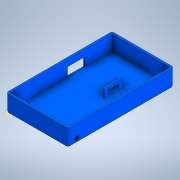
# Autodesk Inventor part: OuterCase
Saved by Autodesk Inventor 2021 (Build 250183000, 183)
## iProperties
Created: 2021-01-18
Part Number: OuterCase
Material: Generic
Document SubType Name: Modeling
Designer: Jayan
Density: 1 g/cm^3
Appearance: Default
Author: Jayan
Autodesk Inventor part; units mm, degrees
ref_plane "YZ Plane" through (0, 0, 0) normal (1, 0, 0) x (0, 1, 0)
ref_plane "XZ Plane" through (0, 0, 0) normal (0, 1, 0) x (-1, 0, 0)
ref_plane "XY Plane" through (0, 0, 0) normal (0, 0, 1) x (1, 0, 0)
sketch "Sketch1" plane through (0, 0, 0) normal (0, 1, 0) x (-1, 0, 0)
  line L0 (0, 0) -> (88.9, 0)
  line L1 (88.9, 0) -> (88.9, -152.4)
  line L2 (88.9, -152.4) -> (0, -152.4)
  line L3 (0, -152.4) -> (0, 0)
  dimension "d0" = 88.9
  dimension "d1" = 152.4
  constraints: 8 end point, 2 parallel, 1 horizontal, 1 perpendicular
  measures "d0" distance of L1.end L2.end
  measures "d1" distance of L0.end L1.end
extrude "Extrusion1" add sketch "Sketch1" along normal blind 25.4
shell "Shell1" thickness 2.54 removed faces 1 at (-59.2667, 25.4, -101.6)
sketch "Sketch2" plane through (-86.36, 2.54, -149.86) normal (1, 0, 0) x (0, 0, -1)
  point P0 (-149.86, -2.54)
sketch "Sketch7" plane through (0, 0, 0) normal (1, 0, 0) x (0, 0, -1)
  line L0 (152.4, 0) -> (0, 0) projected
  line L1 (0, 0) -> (0, 6.35)
  line L2 (0, 0) -> (0, 25.4) projected
  line L3 (0, 6.35) -> (12.7, 6.35)
  dimension "d21" = 6.35
  dimension "d22" = 12.7
  dimension "d23" = 90
  constraints: 4 end point, 1 perpendicular, 1 point on line
  measures "d21" distance of L0.end L1.end
  measures "d22" distance of L1.end L3.end
  measures "d23" angle of L1 L3
hole "Hole1" at (0, 6.35, -12.7) direction (-1, 0, 0) diameter 6.35 depth 2.54 tip angle 118
fillet "Fillet2" radius 3.175 8 edges at (-44.45, 0, 0) (0, 12.7, 0) (0, 0, -76.2) (-88.9, 12.7, 0) (-88.9, 0, -76.2) (-44.45, 0, -152.4) (-88.9, 12.7, -152.4) (0, 12.7, -152.4)
sketch "Sketch9" plane through (-86.36, 2.54, -149.86) normal (1, 0, 0) x (0, 0, -1)
  line L0 (-0.635, 0.635) -> (-0.635, 22.86) projected
  line L1 (-0.635, 0.635) -> (-38.735, 0.635)
  line L2 (0, 0) -> (-147.32, 0) projected
  line L3 (-0.635, 0.635) -> (37.465, 0.635) construction
  line L4 (-38.735, 0.635) -> (-64.135, 0.635)
  line L5 (-64.135, 0.635) -> (-38.735, 0.635)
  line L6 (-38.735, 0.635) -> (-38.735, 13.335)
  line L7 (-38.735, 13.335) -> (-64.135, 13.335)
  line L8 (-64.135, 13.335) -> (-64.135, 0.635)
  point P0 (-149.86, -2.54)
  point P1 (-38.735, 0.635)
  dimension "d39" = 38.1
  dimension "d40" = 180
  dimension "d41" = 25.4
  dimension "d42" = 180
  dimension "d43" = 25.4
  dimension "d44" = 12.7
  constraints: 14 end point, 3 parallel, 2 collinear, 2 horizontal, 1 perpendicular
  measures "d39" distance of L0.start L1.end
  measures "d40" angle of L1 L3
  measures "d41" distance of L1.end L4.end
  measures "d42" angle of L4 L1
  measures "d43" distance of L7.end L6.end
  measures "d44" distance of L6.end L5.end
extrude "Extrusion7" cut sketch "Sketch9" against normal blind 5.08
sketch "Sketch10" plane through (-86.36, 2.54, -149.86) normal (1, 0, 0) x (0, 0, -1)
  line L0 (-38.735, 13.335) -> (-38.735, 0.635) projected
  line L1 (-38.735, 0.635) -> (-64.135, 0.635)
  line L2 (-64.135, 0.635) -> (-64.135, 0)
  line L3 (-64.135, 0) -> (-38.735, 0)
  line L4 (-38.735, 0) -> (-38.735, 0.635)
  point P0 (-149.86, -2.54)
  dimension "d47" = 25.4
  dimension "d48" = 0.635
  constraints: 8 end point, 2 parallel, 1 horizontal, 1 perpendicular
  measures "d47" distance of L3.end L2.end
  measures "d48" distance of L2.end L1.end
extrude "Extrusion8" cut sketch "Sketch10" against normal blind 5.08
sketch "Sketch11" plane through (-86.36, 2.54, -149.86) normal (0, 1, 0) x (1, 0, 0)
  line L0 (0, -64.135) -> (-2.4759, -64.135) projected
  line L1 (0, -64.135) -> (50.8, -64.135)
  line L2 (0, -64.135) -> (50.8, -64.135) construction
  line L3 (50.8, -64.135) -> (53.34, -64.135)
  line L4 (53.34, -64.135) -> (53.34, -38.735)
  line L5 (53.34, -38.735) -> (50.8, -38.735)
  line L6 (50.8, -38.735) -> (50.8, -64.135)
  point P0 (86.36, -149.86)
  dimension "d51" = 50.8
  dimension "d52" = 0
  dimension "d53" = 2.54
  dimension "d54" = 25.4
  constraints: 12 end point, 3 horizontal, 2 parallel, 1 collinear, 1 perpendicular
  measures "d51" distance of L0.start L1.end
  measures "d52" distance between parallel lines of L1 L2
  measures "d53" distance of L5.end L4.end
  measures "d54" distance of L4.end L3.end
extrude "Extrusion9" add sketch "Sketch11" along normal blind 12.7
sketch "Sketch12" plane through (-33.02, 2.54, -85.725) normal (1, 0, 0) x (0, 0, -1)
  line L0 (0, 0) -> (5.08, 0)
  line L1 (25.4, 0) -> (0, 0) projected
  line L2 (0, 0) -> (5.08, 0) construction
  line L3 (25.4, 0) -> (20.32, 0)
  line L4 (25.4, 0) -> (30.48, 0) construction
  line L5 (20.32, 0) -> (20.32, 2.54)
  line L6 (0, 0) -> (25.4, 0) projected
  line L7 (20.32, 0) -> (22.86, 0) construction
  line L8 (20.32, 2.54) -> (5.08, 2.54)
  line L9 (5.08, 2.54) -> (5.08, 8.89)
  line L10 (5.08, 8.89) -> (20.32, 8.89)
  line L11 (20.32, 8.89) -> (20.32, 2.54)
  point P0 (-85.725, -2.54)
  dimension "d57" = 5.08
  dimension "d58" = 0
  dimension "d59" = 5.08
  dimension "d60" = 180
  dimension "d61" = 2.54
  dimension "d62" = 90
  dimension "d63" = 15.24
  dimension "d64" = 6.35
  constraints: 20 end point, 4 horizontal, 3 equal length, 2 collinear, 2 parallel, 2 perpendicular
  measures "d57" distance of L0.start L0.end
  measures "d58" distance between parallel lines of L0 L2
  measures "d59" distance of L1.start L3.end
  measures "d60" angle of L3 L4
  measures "d61" distance of L3.end L5.end
  measures "d62" angle of L7 L5
  measures "d63" distance of L9.end L10.end
  measures "d64" distance of L8.end L9.end
extrude "Extrusion10" cut sketch "Sketch12" against normal blind 12.7
body "Solid1"
